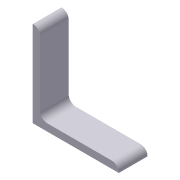
# Autodesk Inventor part: FE-00014-04
Saved by Autodesk Inventor 2012 (Build 160160000, 160)
## iProperties
Company: FIRST
Created: 2008-05-25
Part Number: FE-00014-04
Document SubType Name: Modeling
Designer: dfoster
Density: 1 g/cm^3
Description: Kick Angle
Mass: 23.3711 g
Surface Area: 93.8002 cm^2
Volume: 23.3711 cm^3
Material: Default
Title: Kick Angle
Author: dfoster
Autodesk Inventor part; units mm, degrees
ref_plane "YZ Plane" through (0, 0, 0) normal (1, 0, 0) x (0, 1, 0)
ref_plane "XZ Plane" through (0, 0, 0) normal (0, 1, 0) x (-1, 0, 0)
ref_plane "XY Plane" through (0, 0, 0) normal (0, 0, 1) x (1, 0, 0)
sketch "Sketch1" plane through (0, 0, 0) normal (0, 0, 1) x (1, 0, 0)
  line L0 (-15.875, 68.0517) -> (-15.875, 10.6477)
  line L1 (-9.525, 4.2977) -> (47.879, 4.2977)
  line L2 (53.975, -1.7983) -> (53.975, -2.0523)
  line L3 (53.975, -2.0523) -> (-22.225, -2.0523)
  line L4 (-22.225, -2.0523) -> (-22.225, 74.1477)
  line L5 (-22.225, 74.1477) -> (-21.971, 74.1477)
  arc A0 (-15.875, 68.0517) -> (-21.971, 74.1477) centre (-21.971, 68.0517) ccw
  arc A1 (53.975, -1.7983) -> (47.879, 4.2977) centre (47.879, -1.7983) ccw
  arc A2 (-15.875, 10.6477) -> (-9.525, 4.2977) centre (-9.525, 10.6477) ccw
  dimension "d0" = 6.096
  dimension "d1" = 6.35
  dimension "d2" = 76.2
  dimension "d3" = 6.35
  constraints: 12 end point, 6 point on circle, 6 tangent, 4 parallel, 3 centre point, 3 perpendicular, 1 equal radius
  measures "d0" radius of A0
  measures "d1" distance between parallel lines of L0 L4
  measures "d2" distance of L3.end L4.end
  measures "d3" radius of A2
extrude "Extrusion1" add sketch "Sketch1" along normal blind 25.4
body "Solid1"
